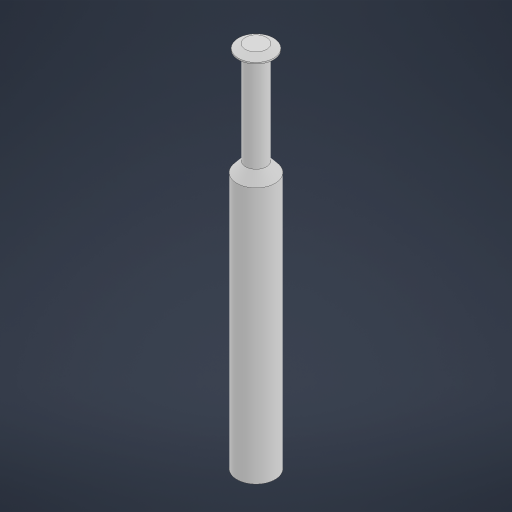
# Autodesk Inventor part: ThreadMillP05-15
Saved by Autodesk Inventor 2024.3 (Build 283343000, 343)
## iProperties
Created: 2024-08-01
Part Number: ThreadMillP05-15
Material: Generic
Document SubType Name: Modeling
Designer: fablabadmin
Density: 1 g/cm^3
Appearance: Default
Author: fablabadmin
Autodesk Inventor part; units mm, degrees
ref_plane "YZ Plane" through (0, 0, 0) normal (1, 0, 0) x (0, 1, 0)
ref_plane "XZ Plane" through (0, 0, 0) normal (0, 1, 0) x (-1, 0, 0)
ref_plane "XY Plane" through (0, 0, 0) normal (0, 0, 1) x (1, 0, 0)
sketch "Sketch1" plane through (0, 0, 0) normal (0, 0, 1) x (1, 0, 0)
  line L0 (0, 0) -> (-2.99, 0)
  line L1 (-2.99, 0) -> (-2.99, 40.4)
  line L2 (-2.99, 40.4) -> (-1.65, 42)
  line L3 (-1.65, 42) -> (-1.65, 56.5)
  line L4 (-1.65, 56.5) -> (-2.76, 57.1409)
  line L5 (-2.949, 57.25) -> (-2.76, 57.3591) construction
  line L6 (-1.65, 58) -> (0, 58)
  line L7 (0, 58) -> (0, 0)
  line L8 (-2.76, 57.3591) -> (-2.76, 57.1409)
  line L9 (-2.76, 57.3591) -> (-1.65, 58)
  line L10 (-2.76, 57.1409) -> (-2.949, 57.25) construction
  dimension "d0" = 58
  dimension "d1" = 5.98
  dimension "d2" = 3.3
  dimension "d3" = 1.5
  dimension "d5" = 16
  dimension "d6" = 1.6
  dimension "d7" = 39.946
  dimension "d8" = 5.52
  dimension "d11" = 1.11
  dimension "d12" = 60
  dimension "d13" = 5.8981
  constraints: 22 end point, 2 collinear, 2 parallel, 2 vertical, 1 equal length, 1 horizontal, 1 perpendicular, 1 point on line
  measures "d0" distance of L6.end L0.start
  measures "d1" diameter of L1 L7
  measures "d2" diameter of L3 L7
  measures "d3" distance of L3.end L6.start
  measures "d5" distance from line of L2.end L6
  measures "d6" vertical distance of L1.end L2.end
  measures "d7" angle of L3 L2
  measures "d8" diameter of L8 L7
  measures "d11" distance from line of L3 L4.end
  measures "d12" angle of L4 L9
  measures "d13" diameter of L5.start L7
revolve "Revolution1" add sketch "Sketch1" angle 360 about axis through (0, 58, 0) along (0, -1, 0)
body "Solid1"
